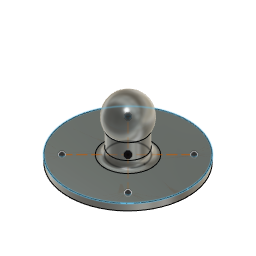
Turntable spool holder knob v1 (Autodesk Fusion 360 design; units mm, degrees)
Autodesk Fusion 360 part; units mm, degrees
note: some values were not read from the file. Set by a fixed rule: which sketch regions a step uses.
sketch "Sketch1" plane through (0, 0, 0) normal (0, 0, 1) x (1, 0, 0)
  line L0 (25, -25) -> (-25, 25) construction
  line L1 (-25, -25) -> (25, 25) construction
  circle A0 centre (0, 0) radius 45
  circle A1 centre (-25, 25) radius 1.525
  circle A2 centre (25, 25) radius 1.525
  circle A3 centre (25, -25) radius 1.525
  circle A4 centre (-25, -25) radius 1.525
  circle A5 centre (0, 0) radius 12.5
  dimension "d1" = 50
  dimension "d2" = 50
  dimension "d3" = 3.05
  dimension "d4" = 3.05
  dimension "d5" = 3.05
  dimension "d6" = 3.05
  dimension "d8" = 25
  constraint coincident L0 A0.centre
  constraint coincident L1 A0.centre
  constraint coincident A0.centre A5.centre
  constraint coincident L0.end A1.centre
  constraint coincident L1.end A2.centre
  constraint coincident L0.start A3.centre
  constraint coincident L1.start A4.centre
  constraint concentric A0 A5
  measures "d1" distance of L0.end L1.end
  measures "d2" distance of L1.start L0.end
  measures "d3" diameter of A1
  measures "d4" diameter of A2
  measures "d5" diameter of A3
  measures "d6" diameter of A4
  measures "d8" diameter of A5
extrude "Extrude1" add sketch "Sketch1" against normal blind 5 contours A0 | A5
extrude "Extrude2" add sketch "Sketch1" along normal blind 25 contours A5
sketch "Sketch2" plane through (0, 0, 25) normal (0, 0, 1) x (-1, 0, 0)
  circle A0 centre (0, 0) radius 12.5
  constraint coincident A0.centre origin
sphere "SpherePrimitive1" add diameter 30 placed x (-1, 0, 0) y (0, -1, 0) z (0, 0, 1) at (0, 0, 25)
fillet "Fillet1" radius 5 1 edges at (-11.6541, 4.5202, 0)
